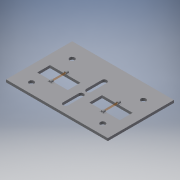
# Autodesk Inventor part: Down
Saved by Autodesk Inventor 2018.1 (Build 221171000, 171)
## iProperties
Created: 2018-12-21
Part Number: Down
Material: Типовые
Document SubType Name: Modeling
Designer: kostya
Density: 1 g/cm^3
Appearance: По умолчанию
Author: kostya
Autodesk Inventor part; units mm, degrees
ref_plane "YZ Plane" through (0, 0, 0) normal (1, 0, 0) x (0, 1, 0)
ref_plane "XZ Plane" through (0, 0, 0) normal (0, 1, 0) x (-1, 0, 0)
sketch "Эскиз1" plane through (0, 0, 0) normal (0, 0, 1) x (1, 0, 0)
  line L0 (-100, -75) -> (100, -75)
  line L1 (100, -75) -> (100, 75)
  line L2 (100, 75) -> (-100, 75)
  line L3 (-100, 75) -> (-100, -75)
  line L4 (-100, -75) -> (100, 75) construction
  line L5 (100, -75) -> (-100, 75) construction
  point P0 (0, 0)
  dimension "d0" = 200
  dimension "d1" = 150
  constraints: 12 end point, 2 midpoint, 2 parallel, 1 horizontal, 1 perpendicular
  measures "d0" distance of L2.end L1.end
  measures "d1" distance of L1.end L0.end
extrude "Выдавливание1" add sketch "Эскиз1" along normal blind 5
sketch "Эскиз2" plane through (0, 0, 5) normal (0, 0, 1) x (1, 0, 0)
  line L0 (-100, -75) -> (100, -75) projected
  line L1 (100, -75) -> (100, 75) projected
  line L2 (100, 75) -> (-100, 75) projected
  line L3 (-100, 75) -> (-100, -75) projected
  line L4 (100, 75) -> (-100, 75) construction
  line L5 (0, 75) -> (0, -75) construction
  line L6 (-100, 0) -> (100, 0) construction
  line L7 (100, -75) -> (100, 75) construction
  line L8 (-100, -12.5) -> (100, -12.5) construction
  line L9 (100, -12.5) -> (100, 12.5) construction
  line L10 (100, 12.5) -> (-100, 12.5) construction
  line L11 (-100, 12.5) -> (-100, -12.5) construction
  line L12 (-100, -12.5) -> (100, 12.5) construction
  line L13 (100, -12.5) -> (-100, 12.5) construction
  line L14 (-100, 0) -> (0, 0) construction
  line L15 (-51.2124, 75) -> (-51.2124, -75) construction
  line L16 (-100, -75) -> (100, -75) construction
  line L17 (0, 0) -> (100, 0) construction
  line L18 (50, 75) -> (50, -75) construction
  line L19 (-81.2124, -12.5) -> (-21.2124, -12.5)
  line L20 (-21.2124, -12.5) -> (-21.2124, 12.5)
  line L21 (-21.2124, 12.5) -> (-81.2124, 12.5)
  line L22 (-81.2124, 12.5) -> (-81.2124, -12.5)
  line L23 (-81.2124, -12.5) -> (-21.2124, 12.5) construction
  line L24 (-21.2124, -12.5) -> (-81.2124, 12.5) construction
  line L25 (81.2124, -12.5) -> (21.2124, -12.5)
  line L26 (21.2124, -12.5) -> (21.2124, 12.5)
  line L27 (21.2124, 12.5) -> (81.2124, 12.5)
  line L28 (81.2124, 12.5) -> (81.2124, -12.5)
  point P0 (-51.2124, 0)
  dimension "d4" = 25
  dimension "d5" = 60
  constraints: 44 end point, 9 midpoint, 6 point on line, 4 parallel, 4 perpendicular, 4 symmetric about line, 2 collinear, 2 horizontal
  measures "d4" distance of L9.end L8.end
  measures "d5" distance of L21.end L20.end
extrude "Выдавливание2" cut sketch "Эскиз2" against normal blind 5 contours L22 L21 L20 L19 | L25 L26 L27 L28
sketch "Эскиз3" plane through (-81.2124, 12.5, 5) normal (0, -1, 0) x (1, 0, 0)
  line L0 (0, 0) -> (60, 0) projected
  line L1 (30, 0) -> (30, 14.9537) construction
  line L2 (30, 0) -> (40, 0) construction
  line L3 (30, 0) -> (35, 0) construction
  line L4 (30, 0) -> (25, 0) construction
  line L5 (25, 0) -> (35, 0) construction
  line L6 (25, 0) -> (35, 0)
  line L7 (30, 0) -> (30, 3) construction
  circle A0 centre (30, 1.5) radius 1.5
  arc A1 (32.3946, 0.7816) -> (27.6054, 0.7816) centre (30, 1.5) ccw
  line L8 (35, 0) -> (32.3946, 0.7816)
  line L9 (25, 0) -> (27.6054, 0.7816)
  point P0 (81.2124, -5)
  dimension "d8" = 10
  dimension "d9" = 5
  dimension "d10" = 5
  dimension "d11" = 3
  dimension "d12" = 1
  constraints: 18 end point, 3 midpoint, 3 point on line, 2 collinear, 2 point on circle, 1 centre point, 1 vertical, 1 vertical alignment, 2 other
  measures "d8" distance of L1.start L2.end
  measures "d9" distance of L1.start L3.end
  measures "d10" distance of L1.start L4.end
  measures "d11" distance of L1.start L7.end
extrude "Выдавливание3" add sketch "Эскиз3" against normal blind 5
mirror "Зеркальное отражение1" about plane through (0, 0, 0) normal (0, 1, 0) of "Выдавливание3"
sketch "Эскиз4" plane through (-81.2124, 12.5, 0) normal (0, -1, 0) x (1, 0, 0)
  circle A0 centre (30, 6.5) radius 1.5 projected
  point P0 (81.2124, 0)
surface extrude "ВыдавПврх1" sketch "Эскиз4" along normal up to next shown yes curves A0
boundary_patch "Участок поверхности1"
boundary_patch "Участок поверхности2"
ref_plane "РабПлоскость1" through (-81.2124, 0, 0) normal (0, -1, 0) x (1, 0, 0)
sketch "Эскиз6" plane through (0, 0, 5) normal (0, 0, 1) x (1, 0, 0)
  line L0 (81.2124, -12.5) -> (21.2124, -12.5) projected
  line L1 (21.2124, -12.5) -> (21.2124, 12.5) projected
  line L2 (21.2124, 12.5) -> (81.2124, 12.5) projected
  line L3 (81.2124, 12.5) -> (81.2124, -12.5) projected
  line L4 (-100, -75) -> (100, -75) projected
  line L5 (100, -75) -> (100, 75) projected
  line L6 (100, 75) -> (-100, 75) projected
  line L7 (-100, 75) -> (-100, -75) projected
  line L8 (-46.2124, -12.5) -> (-46.2124, -17.5) projected
  line L9 (-46.2124, -17.5) -> (-51.2124, -17.5) projected
  line L10 (-51.2124, -17.5) -> (-56.2124, -17.5) projected
  line L11 (-56.2124, -17.5) -> (-56.2124, -12.5) projected
  line L12 (-56.2124, -12.5) -> (-81.2124, -12.5) projected
  line L13 (-81.2124, -12.5) -> (-81.2124, 12.5) projected
  line L14 (-81.2124, 12.5) -> (-56.2124, 12.5) projected
  line L15 (-56.2124, 12.5) -> (-56.2124, 17.5) projected
  line L16 (-56.2124, 17.5) -> (-51.2124, 17.5) projected
  line L17 (-51.2124, 17.5) -> (-46.2124, 17.5) projected
  line L18 (-46.2124, 17.5) -> (-46.2124, 12.5) projected
  line L19 (-46.2124, 12.5) -> (-21.2124, 12.5) projected
  line L20 (-21.2124, 12.5) -> (-21.2124, -12.5) projected
  line L21 (-21.2124, -12.5) -> (-46.2124, -12.5) projected
  line L22 (-100, -75) -> (100, -75) construction
  line L23 (-21.2124, -75) -> (-21.2124, 75) construction
  line L24 (100, 75) -> (-100, 75) construction
  line L25 (-21.2124, 12.5) -> (-21.2124, 75) construction
  line L26 (-21.2124, 75) -> (21.2124, 75) construction
  line L27 (21.2124, 75) -> (21.2124, 12.5) construction
  line L28 (21.2124, 12.5) -> (-21.2124, 12.5) construction
  line L29 (-21.2124, 12.5) -> (-21.2124, 75) construction
  line L30 (-21.2124, -75) -> (21.2124, -75) construction
  line L31 (21.2124, -75) -> (21.2124, -12.5) construction
  line L32 (21.2124, -12.5) -> (-21.2124, -12.5) construction
  line L33 (-21.2124, -12.5) -> (-21.2124, -75) construction
  line L34 (100, -75) -> (100, 75) construction
  line L35 (-100, -7.5) -> (100, -7.5) construction
  line L36 (100, -7.5) -> (100, 7.5) construction
  line L37 (100, 7.5) -> (-100, 7.5) construction
  line L38 (-100, 7.5) -> (-100, -7.5) construction
  line L39 (-100, -7.5) -> (100, 7.5) construction
  line L40 (100, -7.5) -> (-100, 7.5) construction
  line L41 (0, 7.5) -> (0, 17.5) construction
  line L42 (0, -7.5) -> (0, -28.0993) construction
  line L43 (-21.2124, 0) -> (21.2124, 0) construction
  arc A0 (-5, -38.0993) -> (5, -38.0993) centre (0, -38.0993) ccw
  arc A1 (5, -7.5) -> (-5, -7.5) centre (0, -7.5) ccw
  line L44 (-5, -7.5) -> (-5, -38.0993)
  line L45 (5, -38.0993) -> (5, -7.5)
  line L46 (100, 0) -> (-100, 0) construction
  line L47 (-100, 75) -> (-100, -75) construction
  arc A2 (5, 38.0993) -> (-5, 38.0993) centre (0, 38.0993) ccw
  arc A3 (-5, 7.5) -> (5, 7.5) centre (0, 7.5) ccw
  line L48 (-5, 7.5) -> (-5, 38.0993)
  line L49 (5, 38.0993) -> (5, 7.5)
  point P0 (0, 0)
  point P1 (0, -17.7997)
  dimension "d24" = 15
  dimension "d25" = 10
  dimension "d38" = 10
  dimension "d39" = 10
  constraints: 50 end point, 9 midpoint, 8 point on circle, 6 parallel, 6 symmetric about line, 5 point on line, 4 centre point, 4 perpendicular, 3 horizontal, 2 vertical, 1 collinear, 1 tangent, 2 other
  measures "d24" distance of L36.end L35.end
  measures "d25" distance of L41.start L41.end
  measures "d38" diameter of A0
  measures "d39" diameter of A1
extrude "Выдавливание5" cut sketch "Эскиз6" against normal blind 20 contours L44 A1 L45 A0 | L49 A3 L48 A2
mirror "Зеркальное отражение2" about plane through (0, 0, 0) normal (1, 0, 0) of "Выдавливание3", "ВыдавПврх1", "Зеркальное отражение1"
sketch "Эскиз7" plane through (0, 0, 5) normal (0, 0, 1) x (1, 0, 0)
  line L0 (-100, -75) -> (100, -75) projected
  line L1 (100, -75) -> (100, 75) projected
  line L2 (100, 75) -> (-100, 75) projected
  line L3 (-100, 75) -> (-100, -75) projected
  line L4 (-46.2124, -12.5) -> (-46.2124, -17.5) projected
  line L5 (-46.2124, -17.5) -> (-51.2124, -17.5) projected
  line L6 (-51.2124, -17.5) -> (-56.2124, -17.5) projected
  line L7 (-56.2124, -17.5) -> (-56.2124, -12.5) projected
  line L8 (-56.2124, -12.5) -> (-81.2124, -12.5) projected
  line L9 (-81.2124, -12.5) -> (-81.2124, 12.5) projected
  line L10 (-81.2124, 12.5) -> (-56.2124, 12.5) projected
  line L11 (-56.2124, 12.5) -> (-56.2124, 17.5) projected
  line L12 (-56.2124, 17.5) -> (-51.2124, 17.5) projected
  line L13 (-51.2124, 17.5) -> (-46.2124, 17.5) projected
  line L14 (-46.2124, 17.5) -> (-46.2124, 12.5) projected
  line L15 (-46.2124, 12.5) -> (-21.2124, 12.5) projected
  line L16 (-21.2124, 12.5) -> (-21.2124, -12.5) projected
  line L17 (-21.2124, -12.5) -> (-46.2124, -12.5) projected
  line L18 (56.2124, -12.5) -> (56.2124, -17.5) projected
  line L19 (56.2124, -17.5) -> (51.2124, -17.5) projected
  line L20 (51.2124, -17.5) -> (46.2124, -17.5) projected
  line L21 (46.2124, -17.5) -> (46.2124, -12.5) projected
  line L22 (46.2124, -12.5) -> (21.2124, -12.5) projected
  line L23 (21.2124, -12.5) -> (21.2124, 12.5) projected
  line L24 (21.2124, 12.5) -> (46.2124, 12.5) projected
  line L25 (46.2124, 12.5) -> (46.2124, 17.5) projected
  line L26 (46.2124, 17.5) -> (51.2124, 17.5) projected
  line L27 (51.2124, 17.5) -> (56.2124, 17.5) projected
  line L28 (56.2124, 17.5) -> (56.2124, 12.5) projected
  line L29 (56.2124, 12.5) -> (81.2124, 12.5) projected
  line L30 (81.2124, 12.5) -> (81.2124, -12.5) projected
  line L31 (81.2124, -12.5) -> (56.2124, -12.5) projected
  line L32 (-100, 75) -> (-70, 75) construction
  line L33 (-70, 75) -> (-70, 45) construction
  line L34 (-70, 45) -> (-100, 45) construction
  line L35 (-100, 45) -> (-100, 75) construction
  circle A0 centre (-70, 45) radius 5
  line L36 (100, -75) -> (100, 75) construction
  line L37 (100, 0) -> (-100, 0) construction
  line L38 (100, 75) -> (-100, 75) construction
  line L39 (0, 75) -> (0, -75) construction
  line L40 (-100, -75) -> (100, -75) construction
  circle A1 centre (70, 45) radius 5
  line L41 (-100, -75) -> (100, -75) projected
  line L42 (-70, -75) -> (-70, -35) construction
  line L43 (-70, -35) -> (-100, -35) construction
  circle A2 centre (-70, -35) radius 5
  line L44 (70, -75) -> (70, -35) construction
  line L45 (70, -35) -> (100, -35) construction
  circle A3 centre (70, -35) radius 5
  line L46 (-100, -75) -> (-100, -55)
  line L47 (-100, -55) -> (100, -55)
  line L48 (100, -75) -> (100, -55)
  point P0 (0, 0)
  dimension "d30" = 30
  dimension "d31" = 30
  dimension "d32" = 10
  dimension "d35" = 40
  dimension "d36" = 10
  dimension "d37" = 20
  constraints: 26 end point, 6 symmetric about line, 5 perpendicular, 4 centre point, 4 coincident, 4 midpoint, 4 point on line, 2 parallel, 1 horizontal, 2 other
  measures "d30" distance of L33.end L34.end
  measures "d31" distance of L32.end L33.end
  measures "d32" diameter of A0
  measures "d35" distance of L42.start L42.end
  measures "d36" diameter of A2
  measures "d37" distance of L0.start L46.end
extrude "Выдавливание6" cut sketch "Эскиз7" against normal blind 20 contours L3 L47 L1 L0 | A0 | A1 | A2 | A3
body "SRF1"
body "SRF2"
body "SRF3"
body "SRF4"
